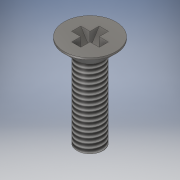
# Autodesk Inventor part: M3x10P
Saved by Autodesk Inventor 2019 (Build 230136000, 136)
## iProperties
Created: 2021-01-02
Part Number: M3x10P
Material: Типовые
Document SubType Name: Modeling
Designer: Professional
Density: 1 g/cm^3
Appearance: С умеренной полировкой
Author: Professional
Autodesk Inventor part; units mm, degrees
ref_plane "YZ Plane" through (0, 0, 0) normal (1, 0, 0) x (0, 1, 0)
ref_plane "XZ Plane" through (0, 0, 0) normal (0, 1, 0) x (-1, 0, 0)
ref_plane "XY Plane" through (0, 0, 0) normal (0, 0, 1) x (1, 0, 0)
sketch "Эскиз1" plane through (0, 0, 0) normal (0, 0, 1) x (1, 0, 0)
  line L0 (-1.4, 0) -> (-1.4, -8.4)
  line L1 (-1.4, -8.4) -> (0, -8.4)
  line L2 (0, -8.4) -> (0, 1.6)
  line L3 (0, 1.6) -> (-2.8, 1.6)
  line L4 (-2.8, 1.6) -> (-2.8, 1.4)
  line L5 (-2.8, 1.4) -> (-1.4, 0)
  point P0 (0, 0)
  dimension "d0" = 2.8
  dimension "d2" = 45
  dimension "d3" = 1.6
  dimension "d4" = 10
  dimension "d5" = 5.6
  constraints: 12 end point, 4 perpendicular, 1 horizontal alignment, 1 point on line, 1 vertical
  measures "d0" diameter of L0 L2
  measures "d2" angle of L2 L5
  measures "d3" distance from line of L0.start L3
  measures "d4" distance between parallel lines of L1 L3
  measures "d5" diameter of L4 L2
revolve "Вращение1" add sketch "Эскиз1" angle 360 about axis through (0, -8.4, 0) along (0, 1, 0)
sketch "Эскиз2" plane through (0, 0, 0) normal (1, 0, 0) x (0, 1, 0)
  line L0 (1.6, -2.8) -> (1.6, 2.8) projected
  line L1 (1.6, 1.5) -> (1.6, 0)
  line L2 (0, 0) -> (1.6, 0)
  line L3 (1.6, 1.5) -> (0, 0.5)
  line L4 (0, -1.4) -> (0, 1.4) projected
  line L5 (0, 0) -> (0, 0.5)
  dimension "d7" = 1.5
  dimension "d13" = 0.5
  constraints: 8 end point, 2 point on line, 1 midpoint, 1 perpendicular, 1 vertical
  measures "d7" distance of L1.start L1.end
  measures "d13" distance from line of L2 L3.end
extrude "Выдавливание1" cut sketch "Эскиз2" along normal mid plane 1
pattern_circular "Круговой массив1" count 4 over 360 about axis through (0, -10, 0) along (0, 1, 0) of "Выдавливание1"
thread "Резьба1" size "M3x0.5" class "6g" standard "ANSI Metric M Profile" full length
